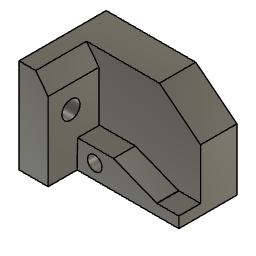
robocon task 1c_1 v1 (Autodesk Fusion 360 design; units mm, degrees)
Autodesk Fusion 360 part; units mm, degrees
sketch "Sketch1" plane through (0, 0, 0) normal (0, 1, 0) x (1, 0, 0)
  line L0 (33.2204, -65) -> (-90, -65)
  line L1 (-90, -65) -> (-90, 65)
  line L2 (-90, 65) -> (90, 65)
  line L3 (90, 65) -> (90, -20)
  line L4 (90, -65) -> (-90, 65) construction
  line L5 (-90, -65) -> (90, 65) construction
  line L6 (33.2204, -65) -> (90, -20)
  constraint horizontal L0
  constraint perpendicular L0 L1
  constraint parallel L0 L2
  constraint parallel L1 L3
  constraint coincident L4 origin
  constraint coincident L5 origin
extrude "Extrude1" add sketch "Sketch1" along normal blind 50 makes body 1
sketch "Sketch2" plane through (0, 0, 0) normal (0, -1, 0) x (1, 0, 0)
  line L0 (33.2204, 65) -> (-90, 65)
  line L1 (-90, 65) -> (-90, -65)
  line L2 (-90, -65) -> (90, -65)
  line L3 (90, -65) -> (90, 20)
  line L4 (90, 20) -> (33.2204, 65)
  line L5 (90, -65) -> (90, -50)
  line L6 (60, -50) -> (0, -26.3208)
  line L7 (0, -26.3208) -> (-50, -26.3208)
  line L8 (-50, -26.3208) -> (-50, -65)
  line L9 (90, -65) -> (90, -50)
  line L10 (60, -50) -> (59.7249, -49.8938)
  line L11 (59.7249, -49.8938) -> (90, -50)
  constraint coincident L2.end L3.start
  constraint coincident L3 L5.end
  constraint perpendicular L2 L5
  constraint perpendicular L5 L7
  constraint coincident L2 L8.end
  constraint perpendicular L2 L8
extrude "Extrude2" add sketch "Sketch2" along normal blind 30 separate body contours L2 L3 L5 L6 L7 L8 L9 L11 makes body 2
sketch "Sketch3" plane through (0, 0, 0) normal (0, -1, 0) x (1, 0, 0)
  line L0 (33.2204, 65) -> (-90, 65)
  line L1 (-90, 65) -> (-90, -65)
  line L2 (-90, -65) -> (90, -65)
  line L3 (90, -65) -> (90, 20)
  line L4 (90, 20) -> (33.2204, 65)
  line L5 (-49.5801, -26.426) -> (-49.5801, 43.0365)
  line L6 (-49.5801, 43.0365) -> (-68.9591, 63.1706)
  line L7 (-68.9591, 63.1706) -> (-90, 63.1706)
  line L8 (-90, -65) -> (-50, -65)
  line L9 (-49.5801, -26.426) -> (-50, -65)
  constraint perpendicular L2 L5
  constraint parallel L0 L7
  constraint coincident L1.end L2.start
  constraint coincident L2 L8.end
  constraint perpendicular L1 L8
extrude "Extrude3" cut sketch "Sketch3" along normal blind 55 contours L1 L2 L5 L6 L7 L8 L9 bodies 2
sketch "Sketch4" plane through (0, 0, 0) normal (0, -1, 0) x (1, 0, 0)
  line L0 (33.2204, 65) -> (-90, 65)
  line L1 (-90, 65) -> (-90, -65)
  line L2 (-90, -65) -> (90, -65)
  line L3 (90, -65) -> (90, 20)
  line L4 (90, 20) -> (33.2204, 65)
  line L5 (-49.2866, -26.0159) -> (-49.2866, 39.6707)
  line L6 (-49.2866, 39.6707) -> (-72.6656, 65)
  line L7 (-71.388, 63.6158) -> (-72.6656, 65)
  line L8 (-90, 65) -> (-90, -65)
  line L9 (-50.1882, -65) -> (-49.2866, -26.0159)
  constraint perpendicular L2 L5
  constraint coincident L0 L6.end
  constraint coincident L6 L7.start
  constraint coincident L0.end L1.start
  constraint coincident L1.end L2.start
  constraint coincident L2 L9.start
extrude "Extrude4" cut sketch "Sketch4" along normal blind 110 contours L0 L1 L2 L5 L6 L7 L8 L9 bodies 2
sketch "Sketch5" plane through (0, 0, 0) normal (0, -1, 0) x (1, 0, 0)
  line L0 (33.2204, 65) -> (-90, 65)
  line L1 (-90, 65) -> (-90, -65)
  line L2 (-90, -65) -> (90, -65)
  line L3 (90, -65) -> (90, 20)
  line L4 (90, 20) -> (33.2204, 65)
  line L5 (-50, -25) -> (-50, 42.5)
  line L6 (-50, 42.5) -> (-67.0234, 65)
  line L7 (-90, 65) -> (-90, -65)
  line L8 (-50, -65) -> (-50, -25)
  constraint vertical L5
  constraint coincident L0 L6.end
  constraint coincident L0.end L1.start
  constraint coincident L1.end L2.start
  constraint coincident L2 L8.start
  constraint perpendicular L2 L8
extrude "Extrude5" add sketch "Sketch5" along normal blind 70 contours L0 L1 L2 L5 L6 L7 L8 bodies 1 2
hole "Hole1" at (-25.7145, -30, -44.8886) direction (0, 1, 0) diameter 20 depth 30 tip angle 118 bodies 1
hole "Hole2" at (-50, -34.8727, 12.4748) direction (-1, 0, 0) diameter 30 depth 30 tip angle 118 bodies 1
delete_face "DeleteFace1" 1 faces at (-60, -33.3792, -2.4506) on bodies 1
hole "Hole3" at (-50, -38.4866, 11.1316) direction (-1, 0, 0) diameter 25 depth 30 tip angle 118 bodies 1
move_face "MoveFace1" to x (1, 0, 0) y (0, 1, 0) z (0, 0, 1) at (15.0004, 0.6456, -1.6309) 1 faces at (-32.4502, 1.3352, -48.7775) on bodies 1
